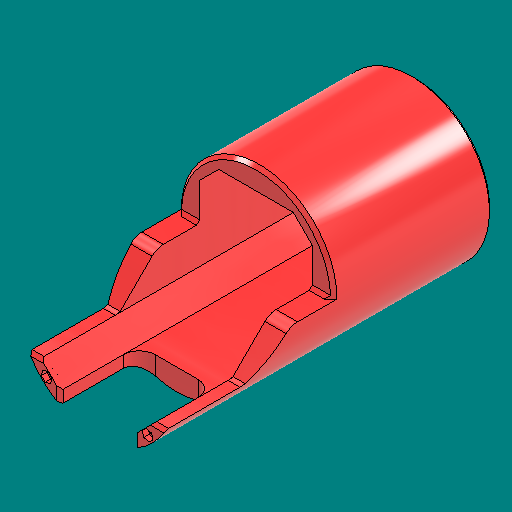
# Autodesk Inventor part: Plasma-Box-Support
Saved by Autodesk Inventor 2025 (Build 290162000, 162)
## iProperties
Created: 2024-06-13
Part Number: Plasma-Box-Support
Material: Generic
Document SubType Name: Modeling
Designer: kuzmin
Density: 1 g/cm^3
Appearance: Light Red
Author: kuzmin
Autodesk Inventor part; units mm, degrees
ref_plane "YZ Plane" through (0, 0, 0) normal (1, 0, 0) x (0, 1, 0)
ref_plane "XZ Plane" through (0, 0, 0) normal (0, 1, 0) x (-1, 0, 0)
ref_plane "XY Plane" through (0, 0, 0) normal (0, 0, 1) x (1, 0, 0)
sketch "Sketch1" plane through (0, 0, 0) normal (0, 0, 1) x (1, 0, 0)
  circle A0 centre (0, 0) radius 52.5
  dimension "d0" = 105
  constraints: 1 centre point, 1 coincident
  measures "d0" diameter of A0
extrude "Extrusion1" add sketch "Sketch1" along normal mid plane 200
sketch "Sketch4" plane through (0, 0, 100) normal (0, 0, 1) x (1, 0, 0)
  line L0 (-35.5, 35.5) -> (35.5, 35.5)
  line L1 (35.5, 35.5) -> (35.5, -35.5)
  line L2 (35.5, -35.5) -> (-35.5, -35.5)
  line L3 (-35.5, -35.5) -> (-35.5, 35.5)
  point P0 (0, 0)
  point P1 (35.5, 0)
  point P2 (0, 35.5)
  dimension "d16" = 71
  constraints: 8 end point, 2 midpoint, 2 parallel, 2 perpendicular, 1 horizontal, 1 horizontal alignment, 1 vertical alignment
  measures "d16" distance of L0.start L0.end
extrude "Extrusion4" cut sketch "Sketch4" against normal through all
chamfer "Chamfer1" distance 12 angle 45 4 edges at (-35.5, 35.5, 0) (-35.5, -35.5, 0) (35.5, -35.5, 0) (35.5, 35.5, 0)
sketch "Sketch5" plane through (0, 0, 100) normal (0, 0, 1) x (1, 0, 0)
  circle A0 centre (0, 0) radius 49
  circle A1 centre (0, 0) radius 52.5 projected
  dimension "d22" = 98
  constraints: 1 centre point, 1 coincident
  measures "d22" diameter of A0
extrude "Extrusion5" cut sketch "Sketch5" against normal through all
sketch "Sketch6" plane through (0, 0, 100) normal (0, 0, 1) x (1, 0, 0)
  circle A0 centre (0, 0) radius 49 projected
  line L0 (-49, 0) -> (49, 0)
  constraints: 2 end point, 2 point on circle, 1 horizontal
extrude "Extrusion6" cut sketch "Sketch6" against normal blind 100 contours L0 A0 picked at (12.7927, 17.7999)
sketch "Sketch7" plane through (0, 0, 100) normal (0, 0, 1) x (1, 0, 0)
  arc A0 (-49, 0) -> (49, 0) centre (0, 0) ccw projected
  line L0 (-35.5, 0) -> (-49, 0) projected
  arc A1 (-49, 0) -> (49, 0) centre (0, 0) ccw projected
  line L1 (49, 0) -> (35.5, 0) projected
  line L2 (35.5, 0) -> (35.5, -23.5) projected
  line L3 (23.5, -35.5) -> (35.5, -23.5) projected
  line L4 (23.5, -35.5) -> (-23.5, -35.5) projected
  line L5 (-35.5, -23.5) -> (-23.5, -35.5) projected
  line L6 (-35.5, -23.5) -> (-35.5, 0) projected
  line L7 (-35.5, -23.5) -> (-42.9971, -23.5)
  line L8 (35.5, -23.5) -> (42.9971, -23.5)
  line L9 (23.5, -35.5) -> (23.5, -42.9971)
  line L10 (-23.5, -35.5) -> (-23.5, -42.9971)
  point P0 (-23.5, -42.9971)
  point P1 (23.5, -42.9971)
  point P2 (42.9971, -23.5)
  point P3 (49, 0)
  point P4 (-42.9971, -23.5)
  constraints: 8 end point, 4 point on circle, 1 horizontal, 1 perpendicular, 1 point on line, 1 vertical
extrude "Extrusion7" cut sketch "Sketch7" against normal blind 50 contours L0 L6 L7 A0 | L10 L4 L9 A0 | L8 L2 L1 A0
chamfer "Chamfer2" distance 23 angle 45 2 edges at (42.25, 0, 50) (-42.25, 0, 50)
fillet "Fillet1" radius 10 2 edges at (-39.2485, -23.5, 50) (39.2485, -23.5, 50)
fillet "Fillet2" radius 10 2 edges at (-23.5, -39.2485, 50) (23.5, -39.2485, 50)
sketch "Sketch8" plane through (0, 0, 100) normal (0, 0, 1) x (1, 0, 0)
  line L0 (31.8198, -31.8198) -> (0, 0) construction
  circle A0 centre (0, 0) radius 45 construction
  line L1 (0, 0) -> (45, 0) construction
  line L2 (49, 0) -> (35.5, 0) projected
  dimension "d34" = 45
  dimension "d35" = 90
  constraints: 4 end point, 2 point on circle, 1 centre point, 1 coincident, 1 point on line
  measures "d34" angle of L0 L1
  measures "d35" diameter of A0
hole "Hole1" at (31.8198, -31.8198, 100) direction (0, 0, -1) diameter 4.4 end through all
sketch "Sketch9" plane through (0, 0, 100) normal (0, 0, 1) x (1, 0, 0)
  circle A0 centre (31.8198, -31.8198) radius 2.2 projected
  line L0 (34.2693, -29.3703) -> (35.1659, -32.7164)
  line L1 (35.1659, -32.7164) -> (32.7164, -35.1659)
  line L2 (32.7164, -35.1659) -> (29.3703, -34.2693)
  line L3 (29.3703, -34.2693) -> (28.4737, -30.9232)
  line L4 (28.4737, -30.9232) -> (30.9232, -28.4737)
  line L5 (30.9232, -28.4737) -> (34.2693, -29.3703)
  line L6 (0, 0) -> (31.8198, -31.8198) construction
  point P0 (29.6985, -29.6985)
  dimension "d46" = 6
  constraints: 14 end point, 1 coincident, 1 midpoint, 1 point on line, 13 other
  measures "d46" distance between parallel lines of L1 L4
extrude "Extrusion8" cut sketch "Sketch9" against normal blind 3.5
pattern_circular "Circular Pattern1" count 2 over 90 about axis through (0, 0, -10) along (0, 0, -1) of "Hole1", "Extrusion8"
mirror "Mirror1" about plane through (0, 0, 0) normal (0, 0, 1) of "Extrusion8", "Hole1", "Circular Pattern1"
chamfer "Chamfer3" distance 2 angle 45 13 edges at (23.5, -39.2485, 100) (39.2485, -23.5, 100) (-23.5, -39.2485, 100) (-39.2485, -23.5, 100) (-42.25, 0, 0) (42.25, 0, 0) (0, 49, 0) (-49, 0, -100) (-29.5, 29.5, -100) (-35.5, 0, -100) (0, 35.5, -100) (29.5, 29.5, -100) (35.5, 0, -100)
fillet "Fillet3" radius 10 2 edges at (42.25, 0, 27) (-42.25, 0, 27)
body "Solid1"
